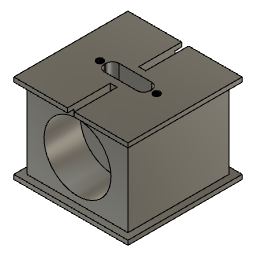
Mag Body 3x1.5 V02 v1 (Autodesk Fusion 360 design; units mm, degrees)
Autodesk Fusion 360 part; units mm, degrees
sketch "Sketch1" plane through (0, 0, 0) normal (0, 0, 1) x (1, 0, 0)
  line L0 (-30.48, 114.973) -> (86.36, 114.973)
  line L1 (86.36, 114.973) -> (86.36, -1.867)
  line L2 (86.36, -1.867) -> (-30.48, -1.867)
  line L3 (-30.48, -1.867) -> (-30.48, 114.973)
  line L4 (1.4449, 65.0493) -> (54.4449, 65.0493)
  line L5 (54.4449, 65.0493) -> (54.4449, 48.0493)
  line L6 (54.4449, 48.0493) -> (1.4449, 48.0493)
  line L7 (1.4449, 48.0493) -> (1.4449, 65.0493)
  line L8 (23.9405, 114.973) -> (31.9405, 114.973)
  line L9 (23.9405, -1.867) -> (31.9405, -1.867)
  line L10 (23.9405, -1.867) -> (31.9405, -1.867)
  line L11 (23.9405, 114.973) -> (31.9405, 114.973)
  dimension "d1" = 116.84
  dimension "d2" = 116.84
  dimension "d3" = 17
  dimension "d4" = 53
  dimension "d5" = 31.9151
  dimension "d8" = 49.9237
  constraint horizontal L0
  constraint vertical L1
  constraint horizontal L2
  constraint vertical L3
  constraint horizontal L4
  constraint vertical L5
  constraint horizontal L6
  constraint vertical L7
  constraint horizontal L8
  constraint coincident L0 L8.start
  constraint horizontal L9
  constraint coincident L2 L9.start
  measures "d1" distance of L0.end L1.end
  measures "d2" distance of L0.start L0.end
  measures "d3" distance of L4.end L5.end
  measures "d4" distance of L5.end L6.end
  measures "d5" distance of L1 L5
  measures "d8" distance of L0 L4
extrude "Extrude1" add sketch "Sketch1" along normal blind 102.616
sketch "Sketch2" plane through (0, -1.867, 0) normal (0, -1, 0) x (1, 0, 0)
  line L0 (-30.48, 0) -> (86.36, 0)
  line L1 (86.36, 102.616) -> (-30.48, 102.616)
  line L2 (-30.48, 102.616) -> (-30.48, 0)
  circle A0 centre (27.94, 51.308) radius 38.735
  line L3 (86.36, 0) -> (86.36, 102.616)
  dimension "d17" = 77.47
  dimension "d18" = 51.308
  dimension "d19" = 58.42
  measures "d17" diameter of A0
  measures "d18" distance of L1 A0.centre
  measures "d19" distance of L2 A0.centre
extrude "Extrude2" cut sketch "Sketch2" against normal blind 42.037 contours A0
sketch "Sketch3" plane through (0, 114.973, 0) normal (0, 1, 0) x (-1, 0, 0)
  line L0 (-86.36, 0) -> (30.48, 0)
  line L1 (30.48, 0) -> (30.48, 102.616)
  line L2 (30.48, 102.616) -> (-86.36, 102.616)
  circle A0 centre (-27.94, 51.308) radius 38.735
  line L3 (-86.36, 102.616) -> (-86.36, 0)
  dimension "d22" = 77.47
  dimension "d23" = 58.42
  dimension "d24" = 51.308
  measures "d22" diameter of A0
  measures "d23" distance of L1 A0.centre
  measures "d24" distance of L2 A0.centre
extrude "Extrude3" cut sketch "Sketch3" against normal blind 42.037 contours A0
sketch "Sketch5" plane through (0, -1.867, 0) normal (0, -1, 0) x (1, 0, 0)
  arc A0 (31.9405, 12.7801) -> (31.9405, 89.8359) centre (27.94, 51.308) ccw
  line L0 (31.9405, 12.7801) -> (31.9405, 0)
  line L1 (31.9405, 0) -> (86.36, 0)
  line L2 (86.36, 0) -> (86.36, 102.616)
  line L3 (86.36, 102.616) -> (31.9405, 102.616)
  line L4 (31.9405, 102.616) -> (31.9405, 89.8359)
  line L5 (86.36, 102.616) -> (86.36, 97.536)
  line L6 (-30.48, 97.536) -> (-30.48, 102.616)
  line L7 (-30.48, 5.08) -> (-30.48, 0)
  line L8 (86.36, 0) -> (86.36, 5.08)
  line L9 (31.9405, 102.616) -> (31.9405, 97.536)
  line L10 (23.9405, 102.616) -> (23.9405, 97.536)
  line L11 (23.9405, 89.836) -> (23.9405, 102.616)
  line L12 (86.36, 97.536) -> (31.9405, 97.536)
  line L13 (23.9405, 97.536) -> (-30.48, 97.536)
  line L14 (-30.48, 102.616) -> (23.9405, 102.616)
  line L15 (31.9405, 102.616) -> (86.36, 102.616)
  line L16 (86.36, 5.08) -> (31.9405, 5.08)
  line L17 (23.9405, 5.08) -> (-30.48, 5.08)
  line L18 (-30.48, 0) -> (23.9405, 0)
  line L19 (31.9405, 0) -> (86.36, 0)
  line L20 (-30.48, 102.616) -> (86.36, 102.616)
  line L21 (23.9405, 5.08) -> (31.9405, 5.08)
  line L22 (23.9405, 0) -> (31.9405, 0)
  dimension "d71" = 5.08
  constraint horizontal L14
  constraint vertical L5
  constraint horizontal L12
  constraint vertical L6
  constraint coincident L2 L5.end
  constraint coincident L3.end L14
  constraint coincident L4 L3.end
  constraint coincident L4 L9.end
  constraint coincident L10.end L12
  constraint perpendicular L10 L12
  constraint coincident L10.start L11
  constraint coincident L17.start L16
  constraint coincident L0 L16.end
  constraint coincident L0 L1.start
  constraint coincident L0.end L18
  constraint collinear L12 L13
  constraint collinear L14 L15
  constraint collinear L16 L17
  constraint collinear L18 L19
  constraint coincident L10.start L20
  constraint coincident L0.end L1.start
  measures "d71" distance of L13 L14
extrude "Extrude5" add sketch "Sketch5" along normal blind 7.62 contours L0 L1 L2 L8 L16 L19 | L0 L7 L17 L18 L21 L22 | L2 L3 L4 L5 L9 L12 L15 L20 | L6 L10 L11 L13 L14 L20
sketch "Sketch6" plane through (86.36, 0, 0) normal (1, 0, 0) x (0, 1, 0)
  line L0 (-1.867, 0) -> (114.973, 0)
  line L1 (114.973, 102.616) -> (-9.487, 102.616)
  line L2 (-9.487, 102.616) -> (-9.487, 97.536)
  line L3 (-9.487, 97.536) -> (-1.867, 97.536)
  line L4 (-9.487, 102.616) -> (114.973, 102.616)
  line L5 (114.973, 102.616) -> (114.973, 97.536)
  line L6 (114.973, 97.536) -> (-9.487, 97.536)
  line L7 (-9.487, 97.536) -> (-9.487, 102.616)
  line L8 (-9.487, 5.08) -> (114.973, 5.08)
  line L9 (114.973, 5.08) -> (114.973, 0)
  line L10 (114.973, 0) -> (-9.487, 0)
  line L11 (-9.487, 0) -> (-9.487, 5.08)
  line L12 (-1.867, 5.08) -> (-9.487, 5.08)
  line L13 (-9.487, 5.08) -> (-9.487, 0)
  line L14 (-9.487, 0) -> (-1.867, 0)
  line L15 (114.973, 0) -> (114.973, 102.616)
  line L16 (-1.867, 97.536) -> (-1.867, 5.08)
  dimension "d54" = 5.08
  dimension "d55" = 5.08
  constraint horizontal L4
  constraint vertical L5
  constraint horizontal L6
  constraint vertical L7
  constraint coincident L1.end L2.start
  constraint horizontal L8
  constraint vertical L9
  constraint horizontal L10
  constraint vertical L11
  constraint coincident L10.end L11.start
  measures "d54" distance of L1.end L2.end
  measures "d55" distance of L8.start L10.end
extrude "Extrude6" add sketch "Sketch6" along normal blind 7.62 contours L0 L8 L9 L10 L11 L12 L13 L14 L15 | L1 L2 L3 L4 L5 L6 L7 L15
sketch "Sketch7" plane through (0, 114.973, 0) normal (0, 1, 0) x (-1, 0, 0)
  line L0 (30.48, 102.616) -> (-93.98, 102.616)
  line L1 (-93.98, 102.616) -> (-93.98, 97.536)
  line L2 (-93.98, 97.536) -> (-86.36, 97.536)
  line L3 (-86.36, 97.536) -> (-86.36, 5.08)
  line L4 (-86.36, 5.08) -> (-93.98, 5.08)
  line L5 (-93.98, 5.08) -> (-93.98, 0)
  line L6 (-93.98, 0) -> (30.48, 0)
  line L7 (30.48, 102.616) -> (30.48, 97.536)
  line L8 (-93.98, 97.536) -> (-93.98, 102.616)
  line L9 (30.48, 0) -> (30.48, 102.616)
  line L10 (30.48, 5.08) -> (30.48, 0)
  line L11 (-93.98, 0) -> (-93.98, 5.08)
  line L12 (-23.9405, 102.616) -> (-23.9405, 97.536)
  line L13 (-23.9405, 89.836) -> (-23.9405, 102.616)
  line L14 (-31.9405, 102.616) -> (-31.9405, 97.536)
  line L15 (-93.98, 5.08) -> (-31.9405, 5.08)
  line L16 (-23.9405, 5.08) -> (30.48, 5.08)
  line L17 (30.48, 0) -> (-23.9405, 0)
  line L18 (-31.9405, 0) -> (-93.98, 0)
  line L19 (-93.98, 102.616) -> (-31.9405, 102.616)
  line L20 (-23.9405, 102.616) -> (30.48, 102.616)
  line L21 (30.48, 97.536) -> (-23.9405, 97.536)
  line L22 (-31.9405, 97.536) -> (-93.98, 97.536)
  circle A0 centre (-27.94, 51.308) radius 38.735
  line L23 (30.48, 0) -> (30.48, 102.616)
  line L24 (-31.9405, 5.08) -> (-23.9405, 5.08)
  line L25 (-31.9405, 0) -> (-23.9405, 0)
  dimension "d58" = 5.08
  dimension "d59" = 5.08
  constraint horizontal L19
  constraint vertical L7
  constraint horizontal L21
  constraint vertical L8
  constraint coincident L0.end L1.start
  constraint coincident L7.end L9
  constraint horizontal L15
  constraint vertical L10
  constraint horizontal L17
  constraint vertical L11
  constraint coincident L9 L6.end
  constraint coincident L4.end L5.start
  constraint coincident L12.start L19
  constraint perpendicular L12 L21
  constraint coincident L12.start L13
  constraint coincident L14.end L21
  constraint coincident L18.start L17
  constraint coincident L16.start L15
  constraint collinear L15 L16
  constraint collinear L17 L18
  constraint collinear L19 L20
  constraint collinear L21 L22
  measures "d58" distance of L0.end L1.end
  measures "d59" distance of L4.end L5.end
extrude "Extrude7" add sketch "Sketch7" along normal blind 7.62 contours L0 L7 L9 L12 L13 L20 L21 L23 | L0 L1 L2 L8 L14 L19 L22 | L4 L5 L6 L9 L10 L11 L15 L16 L17 L18 L23 L24 L25
sketch "Sketch8" plane through (-30.48, 0, 0) normal (-1, 0, 0) x (0, -1, 0)
  line L0 (-122.593, 0) -> (1.867, 0)
  line L1 (1.867, 5.08) -> (1.867, 97.536)
  line L2 (1.867, 97.536) -> (9.487, 97.536)
  line L3 (9.487, 0) -> (9.487, 5.08)
  line L4 (9.487, 102.616) -> (-122.593, 102.616)
  line L5 (-122.593, 102.616) -> (-122.593, 97.536)
  line L6 (-122.593, 97.536) -> (-114.973, 97.536)
  line L7 (-114.973, 97.536) -> (-114.973, 5.08)
  line L8 (-114.973, 5.08) -> (-122.593, 5.08)
  line L9 (-122.593, 5.08) -> (-122.593, 0)
  line L10 (1.867, 0) -> (9.487, 0)
  line L11 (9.487, 5.08) -> (1.867, 5.08)
  line L12 (-122.593, 102.616) -> (9.487, 102.616)
  line L13 (9.487, 102.616) -> (9.487, 97.536)
  line L14 (9.487, 97.536) -> (-122.593, 97.536)
  line L15 (-122.593, 97.536) -> (-122.593, 102.616)
  line L16 (-122.593, 5.08) -> (9.487, 5.08)
  line L17 (9.487, 5.08) -> (9.487, 0)
  line L18 (9.487, 0) -> (-122.593, 0)
  line L19 (-122.593, 0) -> (-122.593, 5.08)
  line L20 (9.487, 97.536) -> (9.487, 102.616)
  constraint horizontal L12
  constraint vertical L13
  constraint horizontal L14
  constraint vertical L15
  constraint coincident L2.end L13.end
  constraint coincident L4.end L5.start
  constraint horizontal L16
  constraint vertical L17
  constraint horizontal L18
  constraint vertical L19
  constraint coincident L3.start L10.end
  constraint coincident L8.end L9.start
sketch "Sketch9" plane through (0, 0, 102.616) normal (0, 0, 1) x (-1, 0, 0)
  line L0 (-54.4449, -48.0493) -> (-1.4449, -48.0493)
  line L1 (-1.4449, -48.0493) -> (-1.4449, -65.0493)
  line L2 (-1.4449, -65.0493) -> (-54.4449, -65.0493)
  line L3 (-54.4449, -65.0493) -> (-54.4449, -48.0493)
  line L4 (-31.9405, -122.593) -> (-31.9405, -114.973)
  line L5 (-23.9405, -114.973) -> (-23.9405, -122.593)
  line L6 (-23.9405, 9.487) -> (-23.9405, 1.867)
  line L7 (-31.9405, 1.867) -> (-31.9405, 9.487)
  circle A0 centre (4.9051, -56.5493) radius 3
  circle A1 centre (-60.7949, -56.5493) radius 3
  line L8 (-23.9405, -122.593) -> (30.48, -122.593)
  line L9 (30.48, 9.487) -> (-23.9405, 9.487)
  line L10 (-31.9405, 9.487) -> (-93.98, 9.487)
  line L11 (-93.98, 9.487) -> (-93.98, -122.593)
  line L12 (-93.98, -122.593) -> (-31.9405, -122.593)
  line L13 (30.48, -122.593) -> (30.48, 9.487)
  line L14 (-23.9405, 1.867) -> (-31.9405, 1.867)
  line L15 (-31.9405, -114.973) -> (-23.9405, -114.973)
  dimension "d64" = 6
  dimension "d65" = 6
  dimension "d67" = 6.35
  dimension "d68" = 8.5
  dimension "d74" = 6.35
  dimension "d75" = 8.5
  measures "d64" diameter of A0
  measures "d65" diameter of A1
  measures "d67" distance of L1 A0.centre
  measures "d68" distance of L2 A1.centre
  measures "d74" distance of L3 A1.centre
  measures "d75" distance of L2 A0.centre
extrude "Extrude9" cut sketch "Sketch9" against normal blind 11 contours A0 | A1
extrude "Extrude10" add sketch "Sketch8" along normal blind 7.62 contours L0 L3 L8 L9 L10 L11 L16 L17 L18 L19 | L2 L4 L5 L6 L12 L13 L14 L15 L20
thread "Thread1" "ANSI Metric M Profile 8.0 M8x1.25 6H" major diameter 8.17 minor diameter 6.7795 pitch 1.25 angle 60 modelled right hand crest width 0.343 on face at (-7.9014, 56.6989, 95.2827) crest through (-8.2949, 56.5493, 102.3035)
thread "Thread2" "ANSI Metric M Profile 8.0 M8x1.25 6H" major diameter 8.17 minor diameter 6.7795 pitch 1.25 angle 60 modelled right hand crest width 0.343 on face at (63.78, 56.848, 95.2827) crest through (57.4051, 56.5493, 102.3035)
fillet "Fillet1" radius 7.62 4 edges at (1.4449, 65.0493, 51.308) (1.4449, 48.0493, 51.308) (54.4449, 65.0493, 51.308) (54.4449, 48.0493, 51.308)
sketch "Sketch10" plane through (0, 0, 102.616) normal (0, 0, 1) x (-1, 0, 0)
  spline S0 degree 3 poles (-61.8528, -60.495) (-62.3436, -60.318) (-62.7957, -60.0483) (-63.5561, -59.3601) (-63.8614, -58.953) (-64.2885, -58.059) (-64.412, -57.5835) (-64.4657, -56.6289) (-64.4018, -56.1595) (-64.1573, -55.4535) (-64.0356, -55.2025) (-63.7383, -54.7403) (-63.5649, -54.53) (-63.3681, -54.3428) knots 0 0 0 0 0.15651 0.15651 0.307908 0.307908 0.454192 0.454192 0.595358 0.595358 0.679011 0.679011 0.76076 0.76076 0.76076 0.76076
  arc A0 (-58.2217, -54.3428) -> (-63.3681, -54.3428) centre (-60.7949, -56.5493) ccw
  spline S1 degree 3 poles (-58.2217, -54.3428) (-57.8975, -54.6513) (-57.6379, -55.0212) (-57.2649, -55.8544) (-57.1612, -56.3122) (-57.1313, -57.2594) (-57.2119, -57.7397) (-57.5559, -58.6599) (-57.8221, -59.0886) (-58.3757, -59.6864) (-58.6166, -59.8906) (-59.1467, -60.2417) (-59.4349, -60.386) (-59.737, -60.495) knots 0 0 0 0 0.134259 0.134259 0.273621 0.273621 0.418082 0.418082 0.567642 0.567642 0.661748 0.661748 0.757764 0.757764 0.757764 0.757764
  arc A1 (-61.8528, -60.495) -> (-59.737, -60.495) centre (-60.7949, -56.5493) ccw
  spline S2 degree 3 poles (3.8472, -60.495) (3.3564, -60.318) (2.9043, -60.0483) (2.1439, -59.3601) (1.8386, -58.953) (1.4115, -58.059) (1.288, -57.5835) (1.2343, -56.6289) (1.2982, -56.1595) (1.5427, -55.4535) (1.6644, -55.2025) (1.9617, -54.7403) (2.1351, -54.53) (2.3319, -54.3428) knots 0 0 0 0 0.15651 0.15651 0.307908 0.307908 0.454192 0.454192 0.595358 0.595358 0.679011 0.679011 0.76076 0.76076 0.76076 0.76076
  arc A2 (7.4783, -54.3428) -> (2.3319, -54.3428) centre (4.9051, -56.5493) ccw
  spline S3 degree 3 poles (7.4783, -54.3428) (7.8025, -54.6513) (8.0621, -55.0212) (8.4351, -55.8544) (8.5388, -56.3122) (8.5687, -57.2594) (8.4881, -57.7397) (8.1441, -58.6599) (7.8779, -59.0886) (7.3243, -59.6864) (7.0834, -59.8906) (6.5533, -60.2417) (6.2651, -60.386) (5.963, -60.495) knots 0 0 0 0 0.134259 0.134259 0.273621 0.273621 0.418082 0.418082 0.567642 0.567642 0.661748 0.661748 0.757764 0.757764 0.757764 0.757764
  arc A3 (3.8472, -60.495) -> (5.963, -60.495) centre (4.9051, -56.5493) ccw
  line L0 (-46.8249, -48.0493) -> (-9.0649, -48.0493)
  arc A4 (-1.4449, -55.6693) -> (-9.0649, -48.0493) centre (-9.0649, -55.6693) ccw
  line L1 (-1.4449, -55.6693) -> (-1.4449, -57.4293)
  arc A5 (-9.0649, -65.0493) -> (-1.4449, -57.4293) centre (-9.0649, -57.4293) ccw
  line L2 (-9.0649, -65.0493) -> (-46.8249, -65.0493)
  arc A6 (-54.4449, -57.4293) -> (-46.8249, -65.0493) centre (-46.8249, -57.4293) ccw
  line L3 (-54.4449, -57.4293) -> (-54.4449, -55.6693)
  arc A7 (-46.8249, -48.0493) -> (-54.4449, -55.6693) centre (-46.8249, -55.6693) ccw
  line L4 (-23.9405, 1.867) -> (-31.9405, 1.867)
  line L5 (-31.9405, 1.867) -> (-31.9405, 9.487)
  line L6 (-31.9405, 9.487) -> (-93.98, 9.487)
  line L7 (-93.98, 9.487) -> (-93.98, -122.593)
  line L8 (-93.98, -122.593) -> (-31.9405, -122.593)
  line L9 (-31.9405, -122.593) -> (-31.9405, -114.973)
  line L10 (-31.9405, -114.973) -> (-23.9405, -114.973)
  line L11 (-23.9405, -114.973) -> (-23.9405, -122.593)
  line L12 (-23.9405, -122.593) -> (38.1, -122.593)
  line L13 (38.1, -122.593) -> (38.1, 9.487)
  line L14 (38.1, 9.487) -> (-23.9405, 9.487)
  line L15 (-23.9405, 9.487) -> (-23.9405, 1.867)
  line L16 (-23.9405, 1.867) -> (-31.9405, 1.867)
  line L17 (-31.9405, 1.867) -> (-31.9405, -40.043)
  line L18 (-31.9405, -40.043) -> (-23.9405, -40.043)
  line L19 (-23.9405, -40.043) -> (-23.9405, 1.867)
  line L20 (-23.9405, -114.973) -> (-31.9405, -114.973)
  line L21 (-31.9405, -114.973) -> (-31.9405, -73.063)
  line L22 (-31.9405, -73.063) -> (-23.9405, -73.063)
  line L23 (-23.9405, -73.063) -> (-23.9405, -114.973)
  dimension "d78" = 41.91
  dimension "d79" = 8
  dimension "d80" = 41.91
  dimension "d81" = 8
  constraint horizontal L16
  constraint vertical L17
  constraint horizontal L18
  constraint vertical L19
  constraint coincident L4.start L15.end
  constraint horizontal L20
  constraint vertical L21
  constraint horizontal L22
  constraint vertical L23
  constraint coincident L10.end L11.start
  measures "d78" distance of L4.start L18.end
  measures "d79" distance of L17.end L18.end
  measures "d80" distance of L10.end L22.end
  measures "d81" distance of L21.end L22.end
extrude "Extrude11" cut sketch "Sketch10" against normal blind 15.24 contours L4 L16 L17 L18 L19 | L10 L20 L21 L22 L23
